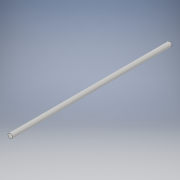
# Autodesk Inventor part: Part13
Saved by Autodesk Inventor 2019 (Build 230136000, 136)
## iProperties
Created: 2021-08-30
Part Number: Part13
Material: 一般
Document SubType Name: Sheet Metal
Designer: yuta
Density: 1 g/cm^3
Sheet Metal Rule: Default_mm
Appearance: 既定
Author: yuta
Autodesk Inventor part; units mm, degrees
ref_plane "YZ Plane" through (0, 0, 0) normal (1, 0, 0) x (0, 1, 0)
ref_plane "XZ Plane" through (0, 0, 0) normal (0, 1, 0) x (-1, 0, 0)
ref_plane "XY Plane" through (0, 0, 0) normal (0, 0, 1) x (1, 0, 0)
sketch "スケッチ1" plane through (0, 0, 0) normal (0, 0, 1) x (1, 0, 0)
  circle A0 centre (-1.0134, 0.6485) radius 1
  point P0 (0, 0)
  dimension "d0" = 2
  constraints: 1 centre point
  measures "d0" diameter of A0
extrude "押し出し1" add sketch "スケッチ1" along normal blind 70
equation "\"BendRadius\" = Thickness"
equation "\"BendReliefWidth\" = Thickness"
equation "\"BendReliefDepth\" = 0.5 * Thickness"
equation "\"CornerReliefSize\" = 4 * Thickness"
equation "\"MinimumRemnant\" = 2 * Thickness"
equation "\"TransitionRadius\" = BendRadius"
equation "\"JacobiRadiusSize\" = BendRadius"
equation "\"GapSize\" = Thickness"
equation "\"Thickness\" = 0.5"
